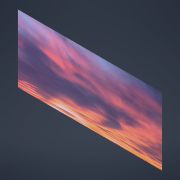
# Autodesk Inventor part: background
Saved by Autodesk Inventor 2022 (Build 260153000, 153)
## iProperties
Created: 2022-02-06
Part Number: background
Material: Generic
Document SubType Name: Modeling
Designer: MatusBarany
Density: 1 g/cm^3
Appearance: Default
Author: MatusBarany
Autodesk Inventor part; units mm, degrees
ref_plane "YZ Plane" through (0, 0, 0) normal (1, 0, 0) x (0, 1, 0)
ref_plane "XZ Plane" through (0, 0, 0) normal (0, 1, 0) x (-1, 0, 0)
ref_plane "XY Plane" through (0, 0, 0) normal (0, 0, 1) x (1, 0, 0)
sketch "Sketch1" plane through (0, 0, 0) normal (0, 0, 1) x (1, 0, 0)
  line L0 (-1381.4803, 769.8415) -> (-1.4803, 769.8415)
  line L1 (-1.4803, 769.8415) -> (-1.4803, 121.8415)
  line L2 (-1.4803, 121.8415) -> (-1381.4803, 121.8415)
  line L3 (-1381.4803, 121.8415) -> (-1381.4803, 769.8415)
  point P0 (0, 0)
  dimension "d0" = 648
  dimension "d1" = 1380
  constraints: 8 end point, 2 parallel, 1 horizontal, 1 perpendicular
  measures "d0" distance of L0.end L1.end
  measures "d1" distance of L1.end L2.end
extrude "Extrusion1" add sketch "Sketch1" along normal blind 1
sketch "Sketch2" plane through (0, 0, 1) normal (0, 0, 1) x (1, 0, 0)
  line L0 (-3815.0031, 7.0011) -> (-1895.4054, 7.0011) construction
  line L1 (-1895.4054, 7.0011) -> (-1895.4054, -1072.7726) construction
  line L2 (-1895.4054, -1072.7726) -> (-3815.0031, -1072.7726) construction
  line L3 (-3815.0031, -1072.7726) -> (-3815.0031, 7.0011) construction
  line L4 (-5084.3881, 1207.0247) -> (-2840.8091, 1207.0247) construction
  line L5 (-2840.8091, 1207.0247) -> (-2840.8091, 85.2352) construction
  line L6 (-2840.8091, 85.2352) -> (-5084.3881, 85.2352) construction
  line L7 (-5084.3881, 85.2352) -> (-5084.3881, 1207.0247) construction
  line L8 (-2516.626, 1231.8236) -> (249.3636, 1217.0808) construction
  line L9 (249.3636, 1217.0808) -> (243.3744, 93.3976) construction
  line L10 (243.3744, 93.3976) -> (-2522.6153, 108.1404) construction
  line L11 (-2522.6153, 108.1404) -> (-2516.626, 1231.8236) construction
  point P0 (0, 0)
  constraints: 6 other
decal "Decal1"
body "Solid1"
